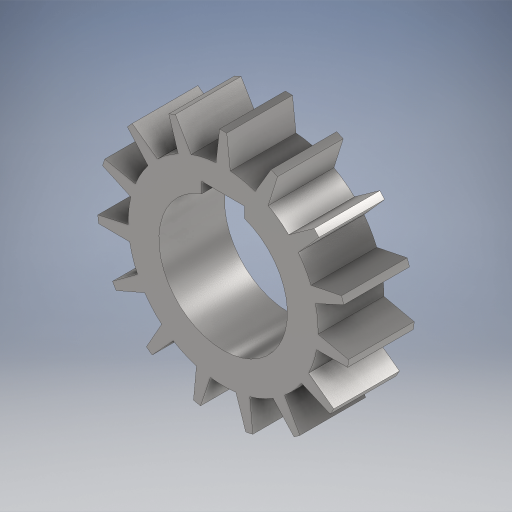
# Autodesk Inventor part: Engranaje pequeño
Saved by Autodesk Inventor 2024.3 (Build 283343010, 343A)
## iProperties
Created: 2025-05-10
Part Number: Engranaje pequeño
Material: Steel, Galvanized
Document SubType Name: Modeling
Designer: Gary
Density: 7.85 g/cm^3
Appearance: Galvanized
Author: Gary
Autodesk Inventor part; units mm, degrees
ref_plane "YZ Plane" through (0, 0, 0) normal (1, 0, 0) x (0, 1, 0)
sketch "Sketch1" plane through (0, 0, 0) normal (0, 0, 1) x (1, 0, 0)
  point P0 (0, 0)
sketch "Sketch2" plane through (0, 0, 0) normal (0, 0, 1) x (1, 0, 0)
  circle A0 centre (0, 0) radius 45
  circle A1 centre (0, 0) radius 66.5
  line L0 (-15, 42.4264) -> (-15, 50)
  line L1 (-15, 50) -> (15, 50)
  line L2 (15, 50) -> (15, 42.4264)
  line L3 (5, 88) -> (5, 87.8578)
  line L4 (0, 88) -> (0, 87.8578)
  line L5 (-5, 66.3118) -> (-2.5041, 87.9644)
  line L6 (5, 66.3118) -> (2.5, 88)
  arc A2 (2.5041, 87.9644) -> (-2.5041, 87.9644) centre (0, 0) ccw
  arc A3 (72.6365, 49.6783) -> (72.4155, 50) centre (0, 0) ccw
  arc A4 (84.4329, 24.8009) -> (82.8853, 29.564) centre (0, 0) ccw
  arc A5 (49.6783, -72.6365) -> (53.73, -69.6928) centre (0, 0) ccw
  arc A6 (-53.73, -69.6928) -> (-49.6783, -72.6365) centre (0, 0) ccw
  arc A7 (-82.8853, 29.564) -> (-84.4329, 24.8009) centre (0, 0) ccw
  line L7 (-31.5392, 58.5451) -> (-38.0659, 79.3409)
  line L8 (-22.4037, 62.6125) -> (-33.509, 81.4088)
  arc A8 (-33.4907, 81.378) -> (-38.0659, 79.3409) centre (0, 0) ccw
  line L9 (-52.6249, 40.6555) -> (-67.0458, 56.9987)
  line L10 (-45.9336, 48.087) -> (-63.7239, 60.7414)
  arc A9 (-63.6947, 60.7206) -> (-67.0458, 56.9987) centre (0, 0) ccw
  line L11 (-64.6113, 15.7362) -> (-84.4329, 24.8009)
  line L12 (-61.5211, 25.2467) -> (-82.9204, 29.5711)
  arc A10 (-82.8853, 29.564) -> (-84.4329, 24.8009) centre (0, 0) ccw
  line L13 (-65.4259, -11.9041) -> (-87.2207, -11.6852)
  line L14 (-66.4711, -1.9589) -> (-87.7792, -6.7122)
  arc A11 (-87.7442, -6.7044) -> (-87.2207, -11.6852) centre (0, 0) ccw
  line L15 (-54.9277, -37.486) -> (-74.9273, -46.1508)
  line L16 (-59.9277, -28.8258) -> (-77.4602, -41.8349)
  arc A12 (-77.4314, -41.8136) -> (-74.9273, -46.1508) centre (0, 0) ccw
  line L17 (-34.932, -56.5863) -> (-49.6783, -72.6365)
  line L18 (-43.0222, -50.7084) -> (-53.7476, -69.724)
  arc A13 (-53.73, -69.6928) -> (-49.6783, -72.6365) centre (0, 0) ccw
  line L19 (-8.8963, -65.9023) -> (-15.8394, -86.5628)
  line L20 (-18.6777, -63.8231) -> (-20.7416, -85.5572)
  arc A14 (-20.7382, -85.5215) -> (-15.8394, -86.5628) centre (0, 0) ccw
  line L21 (18.6777, -63.8231) -> (20.7382, -85.5215)
  line L22 (8.8963, -65.9023) -> (15.8509, -86.5968)
  arc A15 (15.8394, -86.5628) -> (20.7382, -85.5215) centre (0, 0) ccw
  line L23 (43.0222, -50.7084) -> (53.73, -69.6928)
  line L24 (34.932, -56.5863) -> (49.7026, -72.663)
  arc A16 (49.6783, -72.6365) -> (53.73, -69.6928) centre (0, 0) ccw
  line L25 (59.9277, -28.8258) -> (77.4314, -41.8136)
  line L26 (54.9277, -37.486) -> (74.9602, -46.1651)
  arc A17 (74.9273, -46.1508) -> (77.4314, -41.8136) centre (0, 0) ccw
  line L27 (66.4711, -1.9589) -> (87.7442, -6.7044)
  line L28 (65.4259, -11.9041) -> (87.2566, -11.6848)
  arc A18 (87.2207, -11.6852) -> (87.7442, -6.7044) centre (0, 0) ccw
  line L29 (61.5211, 25.2467) -> (82.8853, 29.564)
  line L30 (64.6113, 15.7362) -> (84.4655, 24.8159)
  arc A19 (84.4329, 24.8009) -> (82.8853, 29.564) centre (0, 0) ccw
  line L31 (45.9336, 48.087) -> (63.6947, 60.7206)
  line L32 (52.6249, 40.6555) -> (67.0696, 57.0256)
  arc A20 (67.0458, 56.9987) -> (63.6947, 60.7206) centre (0, 0) ccw
  line L33 (22.4037, 62.6125) -> (33.4907, 81.378)
  line L34 (31.5392, 58.5451) -> (38.0767, 79.3752)
  arc A21 (38.0659, 79.3409) -> (33.4907, 81.378) centre (0, 0) ccw
  point P0 (15, 46.2132)
  point P1 (-15, 46.2132)
  point P2 (5, 77.1559)
  point P3 (0, 77.1559)
  point P4 (0, -88)
  point P5 (-82.8853, 29.564)
  point P6 (-84.4329, 24.8009)
  point P7 (-53.73, -69.6928)
  point P8 (-49.6783, -72.6365)
  point P9 (49.6783, -72.6365)
  point P10 (53.73, -69.6928)
  point P11 (82.8853, 29.564)
  dimension "d2" = 90
  dimension "d3" = 21.5
  dimension "d4" = 30
  dimension "d5" = 50
  dimension "d6" = 88
  dimension "d7" = 15
  dimension "d10" = 38
  dimension "d17" = 360
  constraints: 70 end point, 42 point on circle, 21 centre point, 19 point on line, 5 coincident, 3 parallel, 2 midpoint, 2 perpendicular, 1 vertical, 140 other
  measures "d2" diameter of A0
  measures "d4" distance of point (15, 46.213) point (-15, 46.213)
  measures "d5" distance from line of point (0, 0) L1
  measures "d6" radius of A2
  measures "d7" distance between parallel lines of L4 L2
  measures "d10" distance from line of L4.start L1
extrude "Extrusion1" add sketch "Sketch2" along normal blind 46 contours A1
ref_plane "Work Plane1" through (0, 0, 23) normal (0, 0, 1) x (1, 0, 0)
ref_plane "Work Plane2" through (0, 0, 23) normal (0, 0, 1) x (1, 0, 0)
extrude "Extrusion2" add sketch "Sketch2" along normal blind 46 contours A1 L29 A4 L30 | L27 A18 L28 A1 | A1 L31 A20 L32 | L25 A17 L26 A1 | A1 L33 A21 L34 | L23 A5 L24 A1 | A1 L5 A2 L6 | L21 A15 L22 A1 | A1 L7 A8 L8 | L19 A14 L20 A1 | A1 L9 A9 L10 | L17 A6 L18 A1 | A1 L11 A7 L12 | L15 A12 L16 A1 | A1 L13 A11 L14
body "Solid1"
